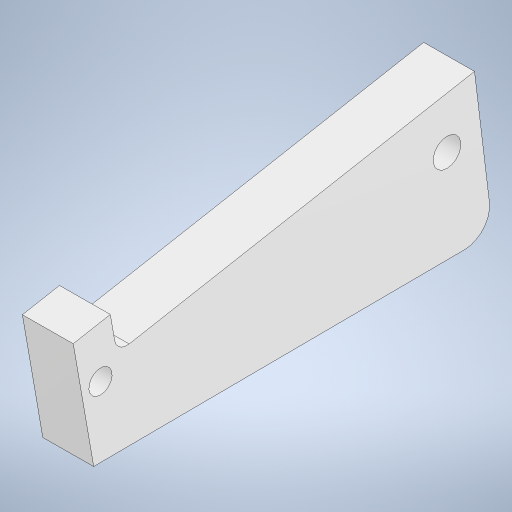
# Autodesk Inventor part: Uprights
Saved by Autodesk Inventor 2023.2 (Build 272271000, 271)
## iProperties
Created: 2024-02-11
Part Number: Uprights
Material: UHMW, White
Document SubType Name: Modeling
Designer: Nathan Cai
Density: 0.94 g/cm^3
Appearance: Smooth - White
Author: Nathan Cai
Autodesk Inventor part; units mm, degrees
ref_plane "YZ Plane" through (0, 0, 0) normal (1, 0, 0) x (0, 1, 0)
ref_plane "XZ Plane" through (0, 0, 0) normal (0, 1, 0) x (-1, 0, 0)
ref_plane "XY Plane" through (0, 0, 0) normal (0, 0, 1) x (1, 0, 0)
sketch "Sketch1" plane through (0, 0, 0) normal (0, 0, 1) x (1, 0, 0)
  line L0 (0, 0) -> (0, 136.525)
  line L1 (-9.6007, 8.6594) -> (-37.7416, 13.6214) construction
  line L2 (-37.7416, 13.6214) -> (-32.2283, 44.8891) construction
  line L3 (-32.2283, 44.8891) -> (-4.0874, 39.9271) construction
  line L4 (-4.0874, 39.9271) -> (-9.6007, 8.6594) construction
  line L5 (-37.7416, 13.6214) -> (-4.0874, 39.9271) construction
  line L6 (-32.2283, 44.8891) -> (-9.6007, 8.6594) construction
  circle A0 centre (-50.8, 12.7) radius 3.175 construction
  circle A1 centre (-50.8, 12.7) radius 6.35 construction
  line L7 (0, 0) -> (-51.5817, 6.3983) construction
  line L8 (-56.5539, 15.3862) -> (0, 136.525) construction
  line L9 (-25.9747, 43.7864) -> (-35.5363, 26.1285) construction
  line L10 (-10.3409, 41.0297) -> (-7.3954, 21.1665) construction
  line L11 (-18.1578, 42.4081) -> (-23.6712, 11.1404) construction
  line L12 (0, 92.075) -> (-19.1732, 95.4558) construction
  line L13 (-32.0394, 9.392) -> (-16.4056, 6.6353) construction
  line L14 (-16.4056, 6.6353) -> (-17.5083, 0.3818) construction
  line L15 (-17.5083, 0.3818) -> (-33.1421, 3.1385) construction
  line L16 (-33.1421, 3.1385) -> (-32.0394, 9.392) construction
  line L17 (-32.0394, 9.392) -> (-38.6124, 4.7896) construction
  line L18 (-16.4056, 6.6353) -> (-12.878, 1.5974) construction
  line L19 (-4.0874, 39.9271) -> (-32.2283, 44.8891) construction
  line L20 (-32.2283, 44.8891) -> (-31.36, 49.8131) construction
  line L21 (-31.36, 49.8131) -> (-3.2192, 44.8511) construction
  line L22 (-3.2192, 44.8511) -> (-4.0874, 39.9271) construction
  line L23 (-50.2487, 15.8268) -> (-50.8, 12.7) construction
  line L24 (-50.8, 12.7) -> (-53.9268, 13.2513) construction
  line L25 (-24.2225, 8.0137) -> (-29.7358, -23.254) construction
  line L26 (-30.3439, 51.0048) -> (-3.7664, 46.3184) construction
  line L27 (-3.7664, 46.3184) -> (-2.9394, 51.0086) construction
  line L28 (-2.9394, 51.0086) -> (-29.5169, 55.6949) construction
  line L29 (-29.5169, 55.6949) -> (-30.3439, 51.0048) construction
  line L30 (-29.9304, 53.3498) -> (-3.3529, 48.6635) construction
  circle A2 centre (-27.5853, 52.9363) radius 1.4732 construction
  circle A3 centre (-21.3318, 51.8337) radius 1.4732 construction
  circle A4 centre (-15.0783, 50.731) radius 1.4732 construction
  circle A5 centre (-8.8248, 49.6284) radius 1.4732
  circle A6 centre (-10.3703, 86.5736) radius 1.4732 construction
  line L31 (-50.8, 12.7) -> (-12.6983, 94.3141) construction
  line L32 (-29.9403, 57.3816) -> (0, 52.1023) construction
  circle A7 centre (-10.3703, 86.5736) radius 4.7625 construction
  line L33 (-4.7625, 52.942) -> (-4.7625, 92.9148) construction
  line L34 (-25.0842, 56.5253) -> (-12.9307, 82.558) construction
  line L35 (-6.6673, 83.5787) -> (-4.7625, 83.2428) construction
  line L36 (-18.6186, 48.9373) -> (-10.8016, 47.5589)
  line L37 (-10.8016, 47.5589) -> (-19.0716, 0.6575)
  line L38 (-19.0716, 0.6575) -> (-26.8885, 2.0358)
  line L39 (-26.8885, 2.0358) -> (-18.6186, 48.9373)
  line L40 (-15.4918, 48.3859) -> (-14.6648, 53.0761)
  line L41 (-14.6648, 53.0761) -> (0, 50.4903)
  circle A8 centre (-11.7154, 5.8083) radius 1.7526
  line L42 (-18.7769, 2.3291) -> (0, 0)
  point P0 (-20.9145, 26.7743)
  point P1 (-17.1994, 2.1334)
  point P2 (-32.9743, 4.0902)
  point P3 (-52.3634, 12.9757)
  point P4 (-48.1138, 18.4539)
  dimension "d13" = 136.525
  dimension "d14" = 31.75
  dimension "d15" = 28.575
  dimension "d16" = 10
  dimension "d17" = 6.35
  dimension "d19" = 50.8
  dimension "d21" = 12.7
  dimension "d22" = 12.7
  dimension "d23" = 7.9375
  dimension "d24" = 19.05
  dimension "d26" = 100
  dimension "d29" = 6.35
  dimension "d30" = 3.175
  dimension "d31" = 7.9375
  dimension "d34" = 5
  dimension "d35" = 26.9875
  dimension "d36" = 3.175
  dimension "d37" = 92.075
  dimension "d38" = 31.75
  dimension "d39" = 41.275
  dimension "d40" = 26.9875
  dimension "d41" = 4.7625
  dimension "d42" = 2.9464
  dimension "d43" = 2.3813
  dimension "d46" = 6.35
  dimension "d51" = 2.9464
  dimension "d52" = 79.7719
  dimension "d53" = 6.35
  dimension "d54" = 9.525
  dimension "d55" = 4.7625
  dimension "d56" = 4.7625
  dimension "d57" = 9.525
  dimension "d58" = 7.9375
  dimension "d59" = 6.35
  dimension "d60" = 4.7625
  dimension "d61" = 3.5052
  dimension "d62" = 12.7
  constraints: 86 end point, 27 point on line, 17 parallel, 9 centre point, 9 perpendicular, 7 midpoint, 6 coincident, 6 point on circle, 2 collinear, 2 tangent, 2 vertical, 11 other
  measures "d13" distance of L0.start L0.end
  measures "d14" distance of L1.end L2.end
  measures "d15" distance between parallel lines of L4 L2
  measures "d16" angle of L0 L4
  measures "d17" diameter of A0
  measures "d19" distance from line of L0 A0.centre
  measures "d21" vertical distance of L0.start A0.centre
  measures "d22" diameter of A1
  measures "d23" distance from line of L9.start L11
  measures "d24" distance from line of L9.end L3
  measures "d26" angle of L0 L12
  measures "d29" distance of L13.end L14.end
  measures "d30" distance between parallel lines of L1 L13
  measures "d31" distance between parallel lines of L14 L11
  measures "d34" distance of L2.end L20.end
  measures "d35" distance between parallel lines of L11 L23
  measures "d36" distance from line of point (-52.363, 12.976) L1
  measures "d37" distance of L0.start point (0, 92.075)
  measures "d38" distance of L25.start L25.end
  measures "d39" distance between parallel lines of L13 L26
  measures "d40" distance between parallel lines of L27 L29
  measures "d41" distance between parallel lines of L26 L28
  measures "d42" diameter of A2
  measures "d43" distance from line of L29 A2.centre
  measures "d46" distance of A2.centre A3.centre
  measures "d51" diameter of A6
  measures "d52" distance from line of L13 A6.centre
  measures "d53" distance between parallel lines of L32 L26
  measures "d54" diameter of A7
  measures "d55" distance between parallel lines of L0 L33
  measures "d56" distance between parallel lines of L31 L34
  measures "d57" distance between parallel lines of L12 L35
  measures "d58" distance of L36.start L36.end
  measures "d59" distance between parallel lines of L11 L37
  measures "d60" distance between parallel lines of L37 L40
  measures "d61" diameter of A8
  measures "d62" distance from line of L11 A8.centre
extrude "Extrusion1" add sketch "Sketch1" along normal blind 6.35 contours L42 L37 L36 L40 L41 L0
fillet "Fillet1" radius 3.175 1 edges at (0, 0, 3.175)
fillet "Fillet4" radius 1.5875 1 edges at (-10.8016, 47.5589, 3.175)
equation "\"d56\" = d55"
body "Solid1"
